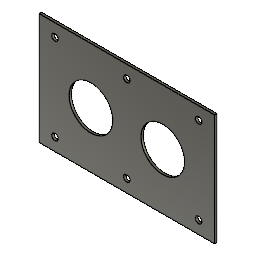
Grande broyeuse v6 (Autodesk Fusion 360 archive; units mm, degrees)
design "cale extérieur"
Autodesk Fusion 360 part; units mm, degrees
sketch "Sketch1" plane through (0, 0, 0) normal (0, 1, 0) x (1, 0, 0)
  line L0 (-88.4437, -50) -> (21.5563, -50)
  line L1 (21.5563, -50) -> (21.5563, 20)
  line L2 (21.5563, 20) -> (-88.4437, 20)
  line L3 (-88.4437, 20) -> (-88.4437, -50)
  line L4 (-88.4437, -15) -> (21.5563, -15) construction
  circle A0 centre (-55.9437, -15) radius 13.6
  circle A1 centre (-10.9437, -15) radius 13.6
  line L5 (-55.9437, -15) -> (-55.9437, -5) construction
  line L6 (-55.9437, -5) -> (-10.9437, -5) construction
  line L7 (-10.9437, -5) -> (-10.9437, -15) construction
  line L8 (-33.4437, -5) -> (-33.4437, -15) construction
  dimension "d1" = 70
  dimension "d2" = 110
  dimension "d3" = 27.2
  dimension "d4" = 45
  constraint horizontal L0
  constraint vertical L1
  constraint horizontal L2
  constraint vertical L3
  constraint midpoint L3 L4.start
  constraint midpoint L1 L4.end
  constraint coincident L4 A0.centre
  constraint coincident L4 A1.centre
  constraint equal A0 A1
  constraint coincident A0.centre L5.start
  constraint perpendicular L4 L5
  constraint perpendicular L5 L6
  constraint perpendicular L6 L7
  constraint coincident A1.centre L7.end
  constraint midpoint L6 L8.start
  constraint perpendicular L6 L8
  constraint midpoint L4 L8.end
  measures "d1" distance of L0.start L2.end
  measures "d2" distance of L0.start L0.end
  measures "d3" diameter of A0
  measures "d4" distance of A0.centre A1.centre L0.start
extrude "Extrude1" add sketch "Sketch1" along normal blind 1.5
sketch "Sketch2" plane through (0, 0, 0) normal (0, -1, 0) x (1, 0, 0)
  circle A0 centre (-10.9437, 15) radius 13.6
  circle A1 centre (-55.9437, 15) radius 13.6
  line L0 (-88.4437, 50) -> (-88.4437, -20)
  line L1 (-88.4437, -20) -> (21.5563, -20)
  line L2 (21.5563, -20) -> (21.5563, 50)
  line L3 (21.5563, 50) -> (-88.4437, 50)
  line L4 (-88.4437, 42) -> (21.5563, 42) construction
  circle A2 centre (-33.4437, 42) radius 2
  circle A3 centre (-78.4437, 42) radius 2
  circle A4 centre (11.5563, 42) radius 2
  line L5 (-88.4437, 15) -> (21.5563, 15) construction
  circle A5 centre (-78.4437, -12) radius 2
  circle A6 centre (-33.4437, -12) radius 2
  circle A7 centre (11.5563, -12) radius 2
  dimension "d7" = 4
  dimension "d8" = 8
  dimension "d9" = 10
  dimension "d10" = 10
  constraint coincident L0 L4.start
  constraint coincident L2 L4.end
  constraint perpendicular L2 L4
  constraint midpoint L4 A2.centre
  constraint coincident L4 A3.centre
  constraint coincident L4 A4.centre
  constraint equal A2 A4
  constraint equal A2 A3
  constraint midpoint L0 L5.start
  constraint midpoint L2 L5.end
  constraint symmetric A2 L5 A6
  constraint symmetric A3 L5 A5
  constraint symmetric A4 L5 A7
  measures "d7" diameter of A3
  measures "d8" distance of L3 L4
  measures "d9" distance of L0 A3.centre
  measures "d10" distance of L2 A4.centre
extrude "Extrude2" cut sketch "Sketch2" against normal through all contours A2 | A3 | A4 | A5 | A6 | A7
equation "d10 = d9"

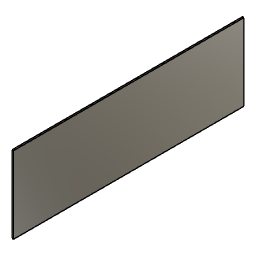
design "Flan"
Autodesk Fusion 360 part; units mm, degrees
sketch "Sketch1" plane through (0, 0, 0) normal (0, 1, 0) x (1, 0, 0)
  line L0 (-8.0856, -31.4139) -> (-6.0856, -31.4139)
  line L1 (-6.0856, -31.4139) -> (-6.0856, 68.5861)
  line L2 (-6.0856, 68.5861) -> (-8.0856, 68.5861)
  line L3 (-8.0856, 68.5861) -> (-8.0856, -31.4139)
  dimension "d7" = 2
  dimension "d8" = 100
  constraint horizontal L0
  constraint vertical L1
  constraint horizontal L2
  constraint vertical L3
  measures "d7" distance of L0.start L0.end
  measures "d8" distance of L0.start L2.end
extrude "Extrude1" add sketch "Sketch1" along normal blind 300

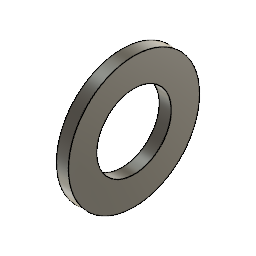
design "rondelle étroite M14 forme Z"
Autodesk Fusion 360 part; units mm, degrees
sketch "Sketch1" plane through (0, 0, 0) normal (1, 0, 0) x (0, 1, 0)
  circle A0 centre (0, 0) radius 7.65
  circle A1 centre (0, 0) radius 13.5
  dimension "d1" = 15.3
  dimension "d2" = 27
  constraint coincident A0.centre A1.centre
  measures "d1" diameter of A0
  measures "d2" diameter of A1
extrude "Extrude1" add sketch "Sketch1" along normal blind 2.5

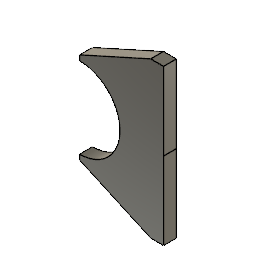
design "entretoise B"
Autodesk Fusion 360 part; units mm, degrees
sketch "Sketch1" plane through (0, 0, 0) normal (0, 1, 0) x (1, 0, 0)
  circle A0 centre (0, 0) radius 14.5 construction
  line L0 (0, -15.6) -> (0, -17.6)
  arc A1 (0, -15.6) -> (15.6, 0) centre (0, 0) ccw
  line L1 (0, -17.6) -> (27.5, -30)
  line L2 (0, 0) -> (15.6, 0) construction
  line L3 (27.5, -30) -> (32.5, -30)
  line L4 (32.5, -30) -> (32.5, 0)
  line L5 (0, -15.6) -> (0, 0) construction
  line L6 (0, 15.6) -> (0, 17.6)
  arc A2 (15.6, 0) -> (0, 15.6) centre (0, 0) ccw
  line L7 (0, 17.6) -> (27.5, 30)
  line L8 (27.5, 30) -> (32.5, 30)
  line L9 (32.5, 30) -> (32.5, 0)
  dimension "d1" = 29
  dimension "d2" = 2
  dimension "d3" = 30
  dimension "d4" = 32.5
  dimension "d5" = 15.6
  dimension "d6" = 5
  constraint coincident A0.centre A1.centre
  constraint horizontal L2
  constraint horizontal L3
  constraint perpendicular L3 L4
  constraint vertical L0
  constraint parallel L0 L5
  constraint symmetric L0.end L2 L6.end
  constraint symmetric L0.start L2 L6.start
  constraint symmetric A1 L2 A2
  constraint symmetric L1.end L2 L7.end
  constraint symmetric L2 A1.end A2.start
  constraint symmetric L2 L3.end L8.end
  constraint symmetric L2 L4.end L9.end
  measures "d1" diameter of A0
  measures "d2" distance of L0.end L0.start
  measures "d3" distance of L2 L3
  measures "d4" distance of A0.centre L4
  measures "d5" radius of A1
  measures "d6" distance of L1.end L3.end
extrude "Extrude1" add sketch "Sketch1" along normal blind 5

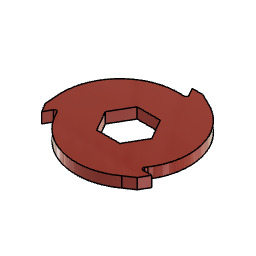
design "Dent A"
Autodesk Fusion 360 part; units mm, degrees
sketch "Sketch1" plane through (0, 0, 0) normal (0, 0, 1) x (1, 0, 0)
  circle A0 centre (0, 0) radius 25
  dimension "d4" = 50
  constraint coincident A0.centre origin
  measures "d4" diameter of A0
extrude "Extrude1" add sketch "Sketch1" along normal blind 5
sketch "Sketch2" plane through (0, 0, 5) normal (0, 0, 1) x (-1, 0, 0)
  circle A0 centre (0, 0) radius 25
  line L0 (5.4848, -9.5) -> (10.9697, 0)
  line L1 (10.9697, 0) -> (5.4848, 9.5)
  line L2 (5.4848, 9.5) -> (-5.4848, 9.5)
  line L3 (-5.4848, 9.5) -> (-10.9697, 0)
  line L4 (-10.9697, 0) -> (-5.4848, -9.5)
  line L5 (-5.4848, -9.5) -> (5.4848, -9.5)
  dimension "d7" = 19
  constraint coincident A0.centre origin
  measures "d7" distance of L0 L3
extrude "Extrude2" cut sketch "Sketch2" against normal through all contours L0 L1 L2 L3 L4 L5
sketch "Sketch3" plane through (0, 0, 5) normal (0, 0, 1) x (-1, 0, 0)
  line L0 (-10.9697, 0) -> (-5.4848, 9.5)
  line L1 (-5.4848, 9.5) -> (5.4848, 9.5)
  line L2 (5.4848, 9.5) -> (10.9697, 0)
  line L3 (10.9697, 0) -> (5.4848, -9.5)
  line L4 (5.4848, -9.5) -> (-5.4848, -9.5)
  line L5 (-5.4848, -9.5) -> (-10.9697, 0)
  circle A0 centre (0, 0) radius 25
  line L6 (0, -9.5) -> (0, -34) construction
  line L7 (0, -30) -> (-3.0461, -24.8137)
  line L8 (0, 0) -> (-21.6506, 12.5) construction
  arc A1 (-21.6506, 12.5) -> (0, -30) centre (1.3758, -2.5344) ccw
  line L9 (0, -30) -> (-5, -30)
  line L10 (-5, -30) -> (-11.5934, -26.7842)
  dimension "d9" = 120
  dimension "d10" = 55
  dimension "d11" = 30
  dimension "d14" = 5
  dimension "d16" = 154
  constraint midpoint L4 L6.start
  constraint perpendicular L4 L6
  constraint coincident L6 L7.start
  constraint coincident A0 L7.end
  constraint coincident A0.centre L8.start
  constraint coincident A0 L8.end
  constraint perpendicular L6 L9
  constraint coincident A1 L10.end
  measures "d9" angle of L6 L8
  measures "d10" diameter of A1
  measures "d11" distance of L7.start A0.centre
  measures "d14" distance of L7.start L9.end
  measures "d16" angle of L9 L10
extrude "Extrude3" add sketch "Sketch3" against normal blind 5 contours A0 L7 A1 L10 | A1 L10 | A1 L9 L10
pattern_circular "C-Pattern1" count 3 over 360 about axis through (0, 0, 1.75) along (0, 0, 1) of "Extrude3"
fillet "Fillet1" radius 1 3 edges at (19.9663, -15.0449, 2.5) (3.0461, 24.8137, 2.5) (-23.0124, -9.7689, 2.5)
sketch "Sketch4" plane through (0, 0, 5) normal (0, 0, 1) x (-1, 0, 0)
  line L0 (-10.9697, 0) -> (-5.4848, 9.5)
  line L1 (-5.4848, 9.5) -> (5.4848, 9.5)
  line L2 (5.4848, 9.5) -> (10.9697, 0)
  line L3 (10.9697, 0) -> (5.4848, -9.5)
  line L4 (5.4848, -9.5) -> (-5.4848, -9.5)
  line L5 (-5.4848, -9.5) -> (-10.9697, 0)
  arc A0 (-1.1597, -24.9731) -> (0, -25) centre (0, 0) ccw
  arc A1 (0, -25) -> (28.8493, 5.3994) centre (1.507, 2.4587) ccw
  line L6 (28.8493, 5.3994) -> (28.4808, 10.6699)
  line L7 (28.4808, 10.6699) -> (25.9808, 15)
  line L8 (25.9808, 15) -> (23.9652, 11.448)
  arc A2 (22.2072, 11.4822) -> (23.9652, 11.448) centre (23.0955, 11.9415) ccw
  arc A3 (22.2072, 11.4822) -> (21.6506, 12.5) centre (0, 0) ccw
  arc A4 (21.6506, 12.5) -> (-19.1007, 22.2845) centre (-2.8828, 0.0758) ccw
  line L9 (-19.1007, 22.2845) -> (-23.4808, 19.3301)
  line L10 (-23.4808, 19.3301) -> (-25.9808, 15)
  line L11 (-25.9808, 15) -> (-21.8968, 15.0305)
  arc A5 (-21.0475, 13.4909) -> (-21.8968, 15.0305) centre (-21.8894, 14.0305) ccw
  arc A6 (-21.0475, 13.4909) -> (-21.6506, 12.5) centre (0, 0) ccw
  arc A7 (-21.6506, 12.5) -> (-9.7486, -27.6839) centre (1.3758, -2.5344) ccw
  line L12 (-9.7486, -27.6839) -> (-5, -30)
  line L13 (-5, -30) -> (0, -30)
  line L14 (0, -30) -> (-2.0683, -26.4785)
  arc A8 (-1.1597, -24.9731) -> (-2.0683, -26.4785) centre (-1.2061, -25.972) ccw
  line L15 (0, 38) -> (0, -40)
  constraint vertical L15
equation "hexa_dent = 19 mm"
equation "hexa_axe = 19 mm"
equation "d7 = hexa_dent"

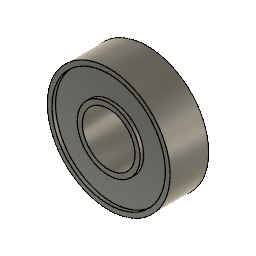
design "Q6202"
Autodesk Fusion 360 part; units mm, degrees
sketch "Sketch1" plane through (0, 0, 0) normal (0, 1, 0) x (1, 0, 0)
  circle A0 centre (0, 0) radius 17.5
  circle A1 centre (0, 0) radius 7.5
  dimension "d1" = 15
  dimension "d2" = 35
  constraint coincident A0.centre A1.centre
  constraint concentric A0 A1
  measures "d1" diameter of A1
  measures "d2" diameter of A0
extrude "Extrude1" add sketch "Sketch1" along normal blind 11
sketch "Sketch2" plane through (0, 0, 0) normal (0, -1, 0) x (1, 0, 0)
  circle A0 centre (0, 0) radius 7.5
  circle A1 centre (0, 0) radius 17.5
  circle A2 centre (0, 0) radius 8.9443
  circle A3 centre (0, 0) radius 16.1245
  constraint concentric A0 A2
  constraint concentric A2 A3
extrude "Extrude2" cut sketch "Sketch2" against normal blind 1 contours A3
ref_plane "WorkPlane1" through (0, 5.5, 0) normal (0, -1, 0) x (-1, 0, 0)
mirror "Mirror1" about plane through (0, 5.5, 0) normal (0, -1, 0) of "Extrude2"

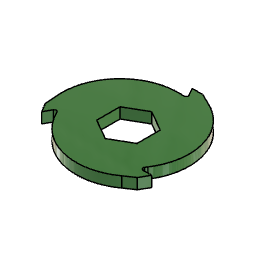
design "Dent B"
Autodesk Fusion 360 part; units mm, degrees
sketch "Sketch1" plane through (0, 0, 0) normal (0, 0, 1) x (1, 0, 0)
  circle A0 centre (0, 0) radius 25
  dimension "d4" = 50
  constraint coincident A0.centre origin
  measures "d4" diameter of A0
extrude "Extrude1" add sketch "Sketch1" along normal blind 5
sketch "Sketch2" plane through (0, 0, 5) normal (0, 0, 1) x (-1, 0, 0)
  circle A0 centre (0, 0) radius 25
  line L0 (9.5, -5.4848) -> (9.5, 5.4848)
  line L1 (9.5, 5.4848) -> (0, 10.9697)
  line L2 (0, 10.9697) -> (-9.5, 5.4848)
  line L3 (-9.5, 5.4848) -> (-9.5, -5.4848)
  line L4 (-9.5, -5.4848) -> (0, -10.9697)
  line L5 (0, -10.9697) -> (9.5, -5.4848)
  dimension "d7" = 19
  constraint coincident A0.centre origin
  measures "d7" distance of L0 L3
extrude "Extrude2" cut sketch "Sketch2" against normal through all contours L0 L1 L2 L3 L4 L5
sketch "Sketch3" plane through (0, 0, 5) normal (0, 0, 1) x (-1, 0, 0)
  line L0 (-9.5, -5.4848) -> (-9.5, 5.4848)
  line L1 (-9.5, 5.4848) -> (0, 10.9697)
  line L2 (0, 10.9697) -> (9.5, 5.4848)
  line L3 (9.5, 5.4848) -> (9.5, -5.4848)
  line L4 (9.5, -5.4848) -> (0, -10.9697)
  line L5 (0, -10.9697) -> (-9.5, -5.4848)
  circle A0 centre (0, 0) radius 25
  line L6 (0, 0) -> (0, -24.1) construction
  line L7 (0, -30) -> (-3.0461, -24.8137)
  line L8 (0, 0) -> (-21.6506, 12.5) construction
  arc A1 (-21.6506, 12.5) -> (0, -30) centre (1.3758, -2.5344) ccw
  line L9 (0, -30) -> (-5, -30)
  line L10 (-5, -30) -> (-11.5934, -26.7842)
  dimension "d9" = 120
  dimension "d10" = 55
  dimension "d11" = 30
  dimension "d14" = 5
  dimension "d16" = 154
  constraint coincident L6 L7.start
  constraint coincident A0 L7.end
  constraint coincident A0.centre L6.start
  constraint coincident A0 L8.end
  constraint perpendicular L6 L9
  constraint coincident A1 L10.end
  measures "d9" angle of L6 L8
  measures "d10" diameter of A1
  measures "d11" distance of L7.start A0.centre
  measures "d14" distance of L7.start L9.end
  measures "d16" angle of L9 L10
extrude "Extrude3" add sketch "Sketch3" against normal blind 5 contours A0 L7 A1 L10 | A1 L10 | A1 L9 L10
pattern_circular "C-Pattern1" count 3 over 360 about axis through (0, 0, 1.75) along (0, 0, 1) of "Extrude3"
fillet "Fillet1" radius 1 3 edges at (19.9663, -15.0449, 2.5) (3.0461, 24.8137, 2.5) (-23.0124, -9.7689, 2.5)
sketch "Sketch4" plane through (0, 0, 5) normal (0, 0, 1) x (-1, 0, 0)
  line L0 (-9.5, -5.4848) -> (-9.5, 5.4848)
  line L1 (-9.5, 5.4848) -> (0, 10.9697)
  line L2 (0, 10.9697) -> (9.5, 5.4848)
  line L3 (9.5, 5.4848) -> (9.5, -5.4848)
  line L4 (9.5, -5.4848) -> (0, -10.9697)
  line L5 (0, -10.9697) -> (-9.5, -5.4848)
  arc A0 (-1.1597, -24.9731) -> (0, -25) centre (0, 0) ccw
  arc A1 (0, -25) -> (28.8493, 5.3994) centre (1.507, 2.4587) ccw
  line L6 (28.8493, 5.3994) -> (28.4808, 10.6699)
  line L7 (28.4808, 10.6699) -> (25.9808, 15)
  line L8 (25.9808, 15) -> (23.9652, 11.448)
  arc A2 (22.2072, 11.4822) -> (23.9652, 11.448) centre (23.0955, 11.9415) ccw
  arc A3 (22.2072, 11.4822) -> (21.6506, 12.5) centre (0, 0) ccw
  arc A4 (21.6506, 12.5) -> (-19.1007, 22.2845) centre (-2.8828, 0.0758) ccw
  line L9 (-19.1007, 22.2845) -> (-23.4808, 19.3301)
  line L10 (-23.4808, 19.3301) -> (-25.9808, 15)
  line L11 (-25.9808, 15) -> (-21.8968, 15.0305)
  arc A5 (-21.0475, 13.4909) -> (-21.8968, 15.0305) centre (-21.8894, 14.0305) ccw
  arc A6 (-21.0475, 13.4909) -> (-21.6506, 12.5) centre (0, 0) ccw
  arc A7 (-21.6506, 12.5) -> (-9.7486, -27.6839) centre (1.3758, -2.5344) ccw
  line L12 (-9.7486, -27.6839) -> (-5, -30)
  line L13 (-5, -30) -> (0, -30)
  line L14 (0, -30) -> (-2.0683, -26.4785)
  arc A8 (-1.1597, -24.9731) -> (-2.0683, -26.4785) centre (-1.2061, -25.972) ccw
  line L15 (0, 31) -> (0, -37)
  constraint vertical L15
equation "hexa_dent = 19 mm"
equation "hexa_axe = 19 mm"
equation "d7 = hexa_dent"

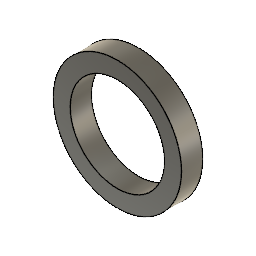
design "entretoise"
Autodesk Fusion 360 part; units mm, degrees
sketch "Sketch1" plane through (0, 0, 0) normal (0, 1, 0) x (1, 0, 0)
  circle A0 centre (0, 0) radius 15
  circle A1 centre (0, 0) radius 11
  dimension "d1" = 30
  dimension "d2" = 22
  constraint coincident A0.centre A1.centre
  measures "d1" diameter of A0
  measures "d2" diameter of A1
extrude "Extrude1" add sketch "Sketch1" along normal blind 5

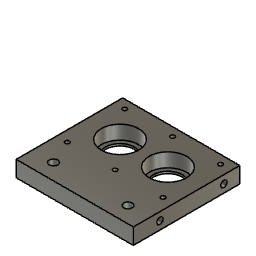
design "Plaque facade A"
Autodesk Fusion 360 part; units mm, degrees
sketch "Sketch1" plane through (0, 0, 0) normal (0, 1, 0) x (1, 0, 0)
  circle A0 centre (-22.5, 0) radius 13.6
  circle A1 centre (22.5, 0) radius 13.6
  line L0 (-22.5, 0) -> (22.5, 0) construction
  line L1 (0, 0) -> (0, -35) construction
  line L2 (-55, -35) -> (55, -35)
  line L3 (55, -35) -> (55, 35)
  line L4 (55, 35) -> (-55, 35)
  line L5 (-55, 35) -> (-55, -35)
  line L6 (-55, 0) -> (-22.5, 0) construction
  dimension "d1" = 27.2
  dimension "d2" = 45
  dimension "d3" = 70
  dimension "d4" = 110
  constraint equal A0 A1
  constraint coincident A0.centre L0.start
  constraint coincident A1.centre L0.end
  constraint horizontal L0
  constraint midpoint L0 L1.start
  constraint perpendicular L0 L1
  constraint coincident L1.start origin
  constraint horizontal L2
  constraint vertical L3
  constraint horizontal L4
  constraint vertical L5
  constraint midpoint L5 L6.start
  constraint perpendicular L5 L6
  constraint midpoint L1.end L2
  measures "d1" diameter of A0
  measures "d2" distance of A0.centre A1.centre
  measures "d3" distance of L2.start L4.end
  measures "d4" distance of L2.start L2.end
extrude "Extrude1" add sketch "Sketch1" along normal blind 15
sketch "Sketch2" plane through (0, 0, 0) normal (0, -1, 0) x (1, 0, 0)
  circle A0 centre (-22.5, 0) radius 13.6
  circle A1 centre (22.5, 0) radius 13.6
  line L0 (-55, 35) -> (-55, -35)
  line L1 (-55, -35) -> (55, -35)
  line L2 (55, -35) -> (55, 35)
  line L3 (55, 35) -> (-55, 35)
  circle A2 centre (-22.5, 0) radius 17.52
  circle A3 centre (22.5, 0) radius 17.52
  dimension "d7" = 35.04
  constraint concentric A0 A2
  constraint concentric A1 A3
  constraint equal A2 A3
  measures "d7" diameter of A2
extrude "Extrude2" cut sketch "Sketch2" against normal blind 13 contours A2 | A3
ref_plane "WorkPlane1" through (0, 7.5, 0) normal (1, 0, 0) x (0, 0, -1)
sketch "Sketch4" plane through (0, 0, 0) normal (0, -1, 0) x (1, 0, 0)
  circle A0 centre (-22.5, 0) radius 17.52
  circle A1 centre (22.5, 0) radius 17.52
  line L0 (-55, 35) -> (-55, -35)
  line L1 (-55, -35) -> (55, -35)
  line L2 (55, -35) -> (55, 35)
  line L3 (55, 35) -> (-55, 35)
  line L4 (-55, 27) -> (55, 27) construction
  circle A2 centre (0, 27) radius 2
  circle A3 centre (-45, 27) radius 2
  circle A4 centre (45, 27) radius 2
  line L5 (55, 0) -> (-55, 0) construction
  circle A5 centre (45, -27) radius 2
  circle A6 centre (0, -27) radius 2
  circle A7 centre (-45, -27) radius 2
  dimension "d16" = 4
  dimension "d17" = 10
  dimension "d18" = 10
  dimension "d20" = 8
  constraint coincident L0 L4.start
  constraint coincident L2 L4.end
  constraint perpendicular L2 L4
  constraint midpoint L4 A2.centre
  constraint coincident L4 A3.centre
  constraint coincident L4 A4.centre
  constraint equal A2 A4
  constraint equal A2 A3
  constraint midpoint L2 L5.start
  constraint midpoint L0 L5.end
  constraint symmetric A2 L5 A6
  constraint symmetric A3 L5 A7
  constraint symmetric A4 L5 A5
  measures "d16" diameter of A3
  measures "d17" distance of L0 A3.centre
  measures "d18" distance of L2 A4.centre
  measures "d20" distance of L3 L4
extrude "Extrude4" cut sketch "Sketch4" against normal through all contours A2 | A3 | A4 | A5 | A6 | A7
move_body "Move1" bodies 1 to x (1, 0, 0) y (0, 0, -1) z (0, 1, 0) at (0, 35, -35)
extrude "Extrude5" add 1 faces at (18.3333, 0, -40) along direction (0, -1, 0) blind 30
sketch "Sketch5" plane through (0, 0, -35) normal (0, 0, 1) x (-1, 0, 0)
  circle A0 centre (0, -62) radius 2
  circle A1 centre (45, -62) radius 2
  circle A2 centre (-45, -62) radius 2
  circle A3 centre (0, -8) radius 2
  circle A4 centre (45, -8) radius 2
  circle A5 centre (-45, -8) radius 2
  circle A6 centre (22.5, -35) radius 17.52
  circle A7 centre (-22.5, -35) radius 17.52
  line L0 (55, -70) -> (55, 30)
  line L1 (55, 30) -> (-55, 30)
  line L2 (-55, 30) -> (-55, -70)
  line L3 (-55, -70) -> (55, -70)
  line L4 (55, 15) -> (-55, 15) construction
  circle A8 centre (35, 15) radius 4
  circle A9 centre (-35, 15) radius 4
  dimension "d23" = 8
  dimension "d24" = 70
  dimension "d25" = 20
  dimension "d26" = 15
  constraint coincident L0 L4.start
  constraint coincident L2 L4.end
  constraint perpendicular L2 L4
  constraint coincident L4 A8.centre
  constraint coincident L4 A9.centre
  constraint equal A8 A9
  measures "d23" diameter of A8
  measures "d24" distance of A8.centre A9.centre
  measures "d25" distance of L2 A9.centre
  measures "d26" distance of L1 L4
extrude "Extrude6" cut sketch "Sketch5" against normal blind 30 contours A8 | A9
sketch "Sketch6" plane through (55, 0, 0) normal (1, 0, 0) x (0, 1, 0)
  line L0 (70, -35) -> (-30, -35)
  line L1 (-30, -35) -> (-30, -50)
  line L2 (-30, -50) -> (70, -50)
  line L3 (70, -50) -> (70, -35)
  line L4 (-30, -42.5) -> (70, -42.5) construction
  circle A0 centre (55, -42.5) radius 3
  circle A1 centre (-5, -42.5) radius 3
  dimension "d30" = 6
  dimension "d31" = 60
  dimension "d32" = 15
  constraint midpoint L1 L4.start
  constraint midpoint L3 L4.end
  constraint coincident L4 A0.centre
  constraint coincident L4 A1.centre
  constraint equal A0 A1
  measures "d30" diameter of A1
  measures "d31" distance of A0.centre A1.centre
  measures "d32" distance of L4.end A0.centre
extrude "Extrude7" cut sketch "Sketch6" against normal blind 20 contours A0 | A1
mirror "Mirror2" about plane through (0, 7.5, 0) normal (1, 0, 0) of "Extrude7"
equation "d25 = ( ( 110 - 70 ) / 2 ) * 1 mm"

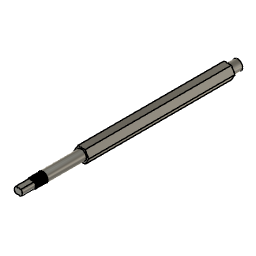
design "axe B"
Autodesk Fusion 360 part; units mm, degrees
sketch "Sketch1" plane through (0, 0, 0) normal (0, 1, 0) x (1, 0, 0)
  line L0 (5.4848, -9.5) -> (10.9697, 0)
  line L1 (10.9697, 0) -> (5.4848, 9.5)
  line L2 (5.4848, 9.5) -> (-5.4848, 9.5)
  line L3 (-5.4848, 9.5) -> (-10.9697, 0)
  line L4 (-10.9697, 0) -> (-5.4848, -9.5)
  line L5 (-5.4848, -9.5) -> (5.4848, -9.5)
  dimension "d1" = 19
  measures "d1" distance of L1 L4
extrude "Extrude1" add sketch "Sketch1" along normal blind 220
sketch "Sketch2" plane through (0, 0, 0) normal (0, -1, 0) x (1, 0, 0)
  line L0 (5.4848, 9.5) -> (-5.4848, 9.5)
  line L1 (-5.4848, 9.5) -> (-10.9697, 0)
  line L2 (-10.9697, 0) -> (-5.4848, -9.5)
  line L3 (-5.4848, -9.5) -> (5.4848, -9.5)
  line L4 (5.4848, -9.5) -> (10.9697, 0)
  line L5 (10.9697, 0) -> (5.4848, 9.5)
  circle A0 centre (0, 0) radius 7.5
  dimension "d4" = 15
  constraint coincident A0.centre origin
  measures "d4" diameter of A0
extrude "Extrude2" add sketch "Sketch2" along normal blind 58 contours A0
sketch "Sketch3" plane through (0, -58, 0) normal (0, -1, 0) x (1, 0, 0)
  circle A0 centre (0, 0) radius 7.5
  circle A1 centre (0, 0) radius 7
  dimension "d7" = 14
  constraint concentric A0 A1
  measures "d7" diameter of A1
extrude "Extrude3" add sketch "Sketch3" along normal blind 17 contours A1
thread "Thread1" "ISO Metric profile 14.0 M14x2 6g" major diameter 13.822 minor diameter 11.534 pitch 2 angle 60 modelled right hand crest width 0.2847 on face at (6.9913, -69.3333, -0.3489) crest through (6.911, -57.5, 0)
sketch "Sketch4" plane through (0, 220, 0) normal (0, 1, 0) x (-1, 0, 0)
  line L0 (5.4848, 9.5) -> (-5.4848, 9.5)
  line L1 (-5.4848, 9.5) -> (-10.9697, 0)
  line L2 (-10.9697, 0) -> (-5.4848, -9.5)
  line L3 (-5.4848, -9.5) -> (5.4848, -9.5)
  line L4 (5.4848, -9.5) -> (10.9697, 0)
  line L5 (10.9697, 0) -> (5.4848, 9.5)
  circle A0 centre (0, 0) radius 7.5
  dimension "d10" = 15
  constraint coincident A0.centre origin
  measures "d10" diameter of A0
extrude "Extrude4" add sketch "Sketch4" along normal blind 15 contours A0
sketch "Sketch5" plane through (0, -75, 0) normal (0, -1, 0) x (1, 0, 0)
  spline S0 degree 3 poles (-3.3483, 4.6955) (-4.0071, 4.3146) (-4.5838, 3.8067) (-5.5311, 2.5793) (-5.8844, 1.8654) (-6.3098, 0.3166) (-6.3676, -0.506) (-6.1666, -2.1557) (-5.8992, -2.9654) (-5.1959, -4.2209) (-4.8371, -4.6975) (-3.9949, -5.5534) (-3.5129, -5.9264) (-2.9883, -6.2315) knots 0 0 0 0 0.228303 0.228303 0.464774 0.464774 0.709409 0.709409 0.962206 0.962206 1.139841 1.139841 1.321288 1.321288 1.321288 1.321288
  arc A0 (-2.9883, -6.2315) -> (2.9883, -6.2315) centre (0, 0) ccw
  spline S1 degree 3 poles (2.9883, -6.2315) (3.7522, -5.7873) (4.4234, -5.2003) (5.482, -3.8207) (5.8675, -3.048) (6.3085, -1.4236) (6.3697, -0.5904) (6.1676, 1.0246) (5.9167, 1.7919) (5.2631, 2.9496) (4.9429, 3.3747) (4.2065, 4.1187) (3.7959, 4.4367) (3.3483, 4.6955) knots 0 0 0 0 0.265106 0.265106 0.522028 0.522028 0.770763 0.770763 1.011307 1.011307 1.170725 1.170725 1.326339 1.326339 1.326339 1.326339
  arc A1 (3.3483, 4.6955) -> (-3.3483, 4.6955) centre (0, 0) ccw
  circle A2 centre (0, 0) radius 6
  dimension "d13" = 12
  constraint coincident A0.centre A1.centre
  measures "d13" diameter of A2
extrude "Extrude5" add sketch "Sketch5" along normal blind 20 contours S0 S1 A1 A2 | S0 S1 A1 A2
sketch "Sketch6" plane through (0, -95, 0) normal (0, -1, 0) x (1, 0, 0)
  circle A0 centre (0, 0) radius 6
  line L0 (0, 0) -> (0, 6) construction
  line L1 (-8, 9.5) -> (10.7231, 9.5)
  line L2 (10.7231, 9.5) -> (10.7231, 4.5)
  line L3 (10.7231, 4.5) -> (-8, 4.5)
  line L4 (-8, 4.5) -> (-8, 9.5)
  line L5 (0, 0) -> (17.434, 0) construction
  line L6 (10.7231, -4.5) -> (-8, -4.5)
  line L7 (-8, -4.5) -> (-8, -9.5)
  line L8 (-8, -9.5) -> (10.7231, -9.5)
  line L9 (10.7231, -9.5) -> (10.7231, -4.5)
  dimension "d16" = 5
  dimension "d17" = 1.5
  constraint coincident A0.centre L0.start
  constraint vertical L0
  constraint horizontal L1
  constraint vertical L2
  constraint horizontal L3
  constraint vertical L4
  constraint coincident A0 L0.end
  constraint perpendicular L0 L5
  constraint symmetric L1.start L5 L7.end
  constraint symmetric L1.end L5 L8.end
  constraint symmetric L2.end L5 L6.start
  constraint symmetric L3.end L5 L6.end
  measures "d16" distance of L1.end L2.end
  measures "d17" distance of L0.end L3
extrude "Extrude6" cut sketch "Sketch6" against normal blind 20 contours A0 L3 | A0 L6
